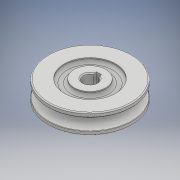
# Autodesk Inventor part: 도면3-3번
Saved by Autodesk Inventor 2018.3 (Build 223284000, 284)
## iProperties
Created: 2019-10-10
Part Number: 도면3-3번
Material: 일반
Document SubType Name: Modeling
Designer: MyTool
Density: 1 g/cm^3
Appearance: 기본값
Author: MyTool
Autodesk Inventor part; units mm, degrees
ref_plane "YZ Plane" through (0, 0, 0) normal (1, 0, 0) x (0, 1, 0)
ref_plane "XZ Plane" through (0, 0, 0) normal (0, 1, 0) x (-1, 0, 0)
ref_plane "XY Plane" through (0, 0, 0) normal (0, 0, 1) x (1, 0, 0)
sketch "스케치1" plane through (0, 0, 0) normal (1, 0, 0) x (0, 1, 0)
  line L0 (0, 0) -> (0, -10)
  line L1 (0, -10) -> (42.5, -10)
  line L2 (42.5, -10) -> (42.5, -5.9758)
  line L3 (42.5, -5.9758) -> (38, -4.6)
  line L4 (38, -4.6) -> (30, -2.1542)
  line L5 (30, -2.1542) -> (30, 0)
  line L6 (30, 0) -> (0, 0)
  dimension "d0" = 38
  dimension "d1" = 17
  dimension "d2" = 4.6
  dimension "d3" = 4.5
  dimension "d4" = 8
  dimension "d5" = 10
  constraints: 14 end point, 3 perpendicular, 2 vertical, 1 point on line
  measures "d0" distance from line of L0 L3.end
  measures "d1" angle of L6 L3
  measures "d2" distance from line of L6 L3.end
  measures "d3" distance from line of L3.end L2
  measures "d4" distance from line of L5 L3.end
  measures "d5" distance between parallel lines of L6 L1
revolve "회전1" add sketch "스케치1" angle 360 about axis through (0, 0, 0) along (0, 0, -1)
fillet "모깎기1" radius 0.5 1 edges at (0, -42.5, -5.9758)
fillet "모깎기2" radius 1 2 edges at (0, -30, -2.1542) (0, -42.5, -10)
sketch "스케치3" plane through (0, 0, -10) normal (0, 0, -1) x (-1, 0, 0)
  circle A0 centre (0, 0) radius 26
  circle A1 centre (0, 0) radius 16
  dimension "d19" = 52
  dimension "d20" = 32
  constraints: 2 centre point, 2 coincident
  measures "d19" diameter of A0
  measures "d20" diameter of A1
extrude "돌출2" cut sketch "스케치3" against normal blind 4
fillet "모깎기4" radius 3 2 edges at (26, 0, -6) (16, 0, -6)
mirror "미러1" about plane through (0, 30, 0) normal (0, 0, 1) of "모깎기2", "회전1", "모깎기1", "돌출2", "모깎기4"
sketch "스케치2" plane through (0, 0, 10) normal (0, 0, 1) x (1, 0, 0)
  circle A0 centre (0, 0) radius 7
  line L0 (-2.5, -3.7) -> (2.5, -3.7)
  line L1 (2.5, -3.7) -> (2.5, 9.3)
  line L2 (2.5, 9.3) -> (-2.5, 9.3)
  line L3 (-2.5, 9.3) -> (-2.5, -3.7)
  point P0 (0, 0)
  dimension "d10" = 14
  dimension "d11" = 2.3
  dimension "d12" = 5
  dimension "d13" = 2.5
  constraints: 8 end point, 2 parallel, 1 centre point, 1 coincident, 1 horizontal, 1 perpendicular
  measures "d10" diameter of A0
  measures "d11" distance edge to line of A0 L2
  measures "d12" distance between parallel lines of L1 L3
  measures "d13" distance from line of point (0, 0) L3
extrude "돌출1" cut sketch "스케치2" against normal up to next
chamfer "모따기1" distance 1 angle 45 2 edges at (0, -7, 10) (0, -7, -10)
